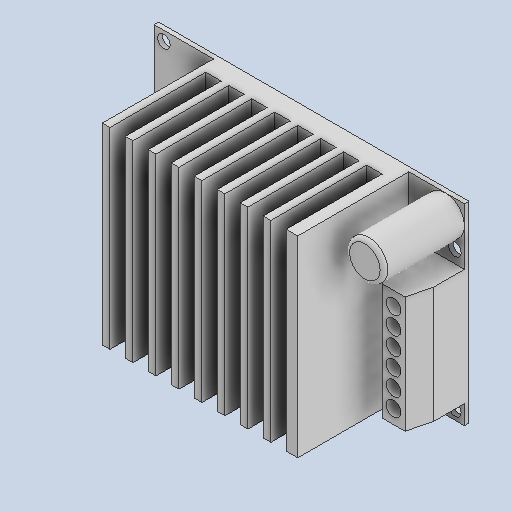
# Autodesk Inventor part: HiLetgoTB6600HG
Saved by Autodesk Inventor 2025.2 (Build 292293000, 293)
## iProperties
Created: 2025-02-08
Part Number: HiLetgoTB6600HG
Material: Generic
Document SubType Name: Modeling
Designer: LattePanda
Density: 1 g/cm^3
Appearance: Default
Author: LattePanda
Autodesk Inventor part; units mm, degrees
ref_plane "YZ Plane" through (0, 0, 0) normal (1, 0, 0) x (0, 1, 0)
ref_plane "XZ Plane" through (0, 0, 0) normal (0, 1, 0) x (-1, 0, 0)
ref_plane "XY Plane" through (0, 0, 0) normal (0, 0, 1) x (1, 0, 0)
sketch "Sketch1" plane through (0, 0, 0) normal (0, 0, 1) x (1, 0, 0)
  line L0 (-40.485, -25.075) -> (40.485, -25.075)
  line L1 (40.485, -25.075) -> (40.485, 25.075)
  line L2 (40.485, 25.075) -> (-40.485, 25.075)
  line L3 (-40.485, 25.075) -> (-40.485, -25.075)
  line L4 (-40.485, -25.075) -> (40.485, 25.075) construction
  line L5 (40.485, -25.075) -> (-40.485, 25.075) construction
  circle A0 centre (-37.975, 22.565) radius 1.65
  line L6 (-39.625, 24.215) -> (-36.325, 24.215) construction
  line L7 (-36.325, 24.215) -> (-36.325, 20.915) construction
  line L8 (-36.325, 20.915) -> (-39.625, 20.915) construction
  line L9 (-39.625, 20.915) -> (-39.625, 24.215) construction
  line L10 (-39.625, 24.215) -> (-36.325, 20.915) construction
  line L11 (-36.325, 24.215) -> (-39.625, 20.915) construction
  line L12 (-40.485, 0) -> (40.485, 0) construction
  line L13 (0, 25.075) -> (0, -25.075) construction
  circle A1 centre (-37.975, -22.565) radius 1.65
  line L14 (0, -25.075) -> (0, 25.075) construction
  circle A2 centre (37.975, 22.565) radius 1.65 construction
  circle A3 centre (37.975, -22.565) radius 1.65
  line L15 (37.975, 25.075) -> (37.975, 13.575) construction
  circle A4 centre (37.975, 13.575) radius 1.65
  point P0 (0, 0)
  dimension "d0" = 80.97
  dimension "d1" = 50.15
  dimension "d2" = 3.3
  dimension "d3" = 0.86
  dimension "d4" = 0.86
  dimension "d10" = 11.5
  constraints: 32 end point, 8 midpoint, 5 centre point, 5 symmetric about line, 4 parallel, 2 horizontal, 2 perpendicular, 2 tangent, 1 coincident, 1 equal radius, 1 point on line, 1 vertical, 3 other
  measures "d0" distance of L1.end L2.end
  measures "d1" distance of L2.end L0.start
  measures "d2" diameter of A0
  measures "d3" distance between parallel lines of L2 L6
  measures "d4" distance between parallel lines of L3 L9
  measures "d10" distance of L15.start L15.end
extrude "Extrusion1" add sketch "Sketch1" along normal blind 1.17
sketch "Sketch2" plane through (0, 0, 1.17) normal (0, 0, 1) x (1, 0, 0)
  line L0 (40.485, -25.075) -> (40.485, 25.075) projected
  line L1 (40.485, -20.075) -> (30.485, -20.075)
  line L2 (30.485, -20.075) -> (30.485, 10.275)
  line L3 (30.485, 10.275) -> (40.485, 10.275)
  line L4 (40.485, 10.275) -> (40.485, -20.075)
  line L5 (-40.485, -25.075) -> (40.485, -25.075) projected
  point P0 (0, 0)
  dimension "d7" = 5
  dimension "d8" = 30.35
  dimension "d9" = 10
  constraints: 8 end point, 2 parallel, 1 horizontal, 1 perpendicular, 1 point on line
  measures "d7" distance between parallel lines of L5 L1
  measures "d8" distance of L1.end L2.end
  measures "d9" distance between parallel lines of L0 L2
extrude "Extrusion2" add sketch "Sketch2" along normal blind 14
sketch "Sketch3" plane through (0, 0, 1.17) normal (0, 0, 1) x (1, 0, 0)
  line L0 (40.485, 10.275) -> (40.485, 25.075) construction
  line L1 (40.485, 25.075) -> (-40.485, 25.075) construction
  circle A0 centre (35.485, 20.075) radius 5
  point P0 (0, 0)
  dimension "d13" = 10
  constraints: 2 tangent, 1 centre point
  measures "d13" diameter of A0
extrude "Extrusion3" add sketch "Sketch3" along normal blind 21
fillet "Fillet1" radius 1 1 edges at (30.485, 20.075, 22.17)
sketch "Sketch4" plane through (30.485, -20.075, 1.17) normal (0, -1, 0) x (1, 0, 0)
  line L0 (0, 14) -> (10, 14) construction
  line L1 (0, 0) -> (0, 14) projected
  line L2 (10, 0) -> (10, 14) projected
  line L3 (10, 14) -> (0, 14) projected
  line L4 (2.5, 14) -> (8.5, 14)
  line L5 (10, 8) -> (8.5, 14)
  line L6 (2.5, 14) -> (0, 8)
  line L7 (10, 8) -> (0, 8) construction
  point P0 (-30.485, -1.17)
  dimension "d17" = 6
  dimension "d18" = 6
  dimension "d19" = 1.5
  constraints: 8 end point, 4 point on line, 1 horizontal
  measures "d17" distance between parallel lines of L7 L0
  measures "d18" distance of L4.end L4.start
  measures "d19" distance of L0.end L4.end
extrude "Extrusion4" cut sketch "Sketch4" against normal up to surface (30.35 mm away)
sketch "Sketch5" plane through (0, 0, 15.17) normal (0, 0, 1) x (1, 0, 0)
  line L0 (38.985, 10.275) -> (32.985, 10.275) construction
  line L1 (35.985, 10.275) -> (35.985, -20.075) construction
  line L2 (32.985, -20.075) -> (38.985, -20.075) construction
  line L3 (35.985, -20.075) -> (35.985, 10.275) construction
  circle A0 centre (35.985, 6.6536) radius 1.925
  circle A1 centre (35.985, 2.0321) radius 1.925
  circle A2 centre (35.985, -2.5893) radius 1.925
  circle A3 centre (35.985, -7.2107) radius 1.925
  circle A4 centre (35.985, -11.8321) radius 1.925
  circle A5 centre (35.985, -16.4536) radius 1.925
  point P0 (0, 0)
  dimension "d22" = 3.85
  dimension "d23" = 4.6214
  dimension "d24" = 4.6214
  dimension "d25" = 4.6214
  dimension "d26" = 4.6214
  dimension "d27" = 4.6214
  dimension "d28" = 3.6214
  dimension "d29" = 3.6214
  constraints: 6 centre point, 6 point on line, 5 equal radius, 4 end point, 2 midpoint, 1 collinear
  measures "d22" diameter of A0
  measures "d23" distance of A1.centre A0.centre
  measures "d24" distance of A2.centre A1.centre
  measures "d25" distance of A3.centre A2.centre
  measures "d26" distance of A4.centre A3.centre
  measures "d27" distance of A4.centre A5.centre
  measures "d28" distance from line of A0.centre L0
  measures "d29" distance from line of L2 A5.centre
extrude "Extrusion5" cut sketch "Sketch5" against normal blind 3.85
sketch "Sketch6" plane through (0, 0, 1.17) normal (0, 0, 1) x (1, 0, 0)
  line L0 (-25.015, 25.075) -> (25.985, 25.075)
  line L1 (25.985, 25.075) -> (25.985, -25.075)
  line L2 (25.985, -25.075) -> (-25.015, -25.075)
  line L3 (-25.015, -25.075) -> (-25.015, 25.075)
  line L4 (40.485, -25.075) -> (40.485, -20.075) projected
  line L5 (35.485, 25.075) -> (-40.485, 25.075) projected
  line L6 (-40.485, -25.075) -> (40.485, -25.075) projected
  point P0 (0, 0)
  dimension "d32" = 14.5
  dimension "d33" = 51
  constraints: 8 end point, 2 collinear, 2 parallel, 1 horizontal, 1 perpendicular
  measures "d32" distance between parallel lines of L4 L1
  measures "d33" distance between parallel lines of L1 L3
extrude "Extrusion6" add sketch "Sketch6" along normal blind 29
sketch "Sketch7" plane through (0, 0, 30.17) normal (0, 0, 1) x (1, 0, 0)
  line L0 (25.985, 25.075) -> (-25.015, 25.075) projected
  line L1 (-25.015, -25.075) -> (25.985, -25.075) projected
  line L2 (22.985, 25.075) -> (18.985, 25.075)
  line L3 (18.985, 25.075) -> (18.985, -25.075)
  line L4 (18.985, -25.075) -> (22.985, -25.075)
  line L5 (22.985, -25.075) -> (22.985, 25.075)
  line L6 (25.985, -25.075) -> (25.985, 25.075) projected
  line L7 (16.985, 25.075) -> (16.985, -25.075)
  line L8 (12.985, 25.075) -> (12.985, -25.075)
  line L9 (10.985, 25.075) -> (10.985, -25.075)
  line L10 (6.985, 25.075) -> (6.985, -25.075)
  line L11 (4.985, 25.075) -> (4.985, -25.075)
  line L12 (0.985, 25.075) -> (0.985, -25.075)
  line L13 (-1.015, 25.075) -> (-1.015, -25.075)
  line L14 (-5.015, 25.075) -> (-5.015, -25.075)
  line L15 (-7.015, 25.075) -> (-7.015, -25.075)
  line L16 (-11.015, 25.075) -> (-11.015, -25.075)
  line L17 (-13.015, 25.075) -> (-13.015, -25.075)
  line L18 (-17.015, 25.075) -> (-17.015, -25.075)
  line L19 (-19.015, 25.075) -> (-19.015, -25.075)
  line L20 (-23.015, 25.075) -> (-23.015, -25.075)
  point P0 (0, 0)
  dimension "d36" = 3
  dimension "d37" = 4
  dimension "d38" = 2
  dimension "d39" = 4
  dimension "d40" = 2
  dimension "d41" = 4
  dimension "d42" = 2
  dimension "d43" = 4
  dimension "d44" = 2
  dimension "d45" = 4
  dimension "d46" = 2
  dimension "d47" = 4
  dimension "d48" = 2
  dimension "d49" = 4
  dimension "d50" = 2
  dimension "d51" = 4
  constraints: 36 end point, 12 vertical, 4 parallel, 1 horizontal, 1 perpendicular, 32 other
  measures "d36" distance between parallel lines of L6 L5
  measures "d37" distance between parallel lines of L5 L3
  measures "d38" distance between parallel lines of L3 L7
  measures "d39" distance between parallel lines of L7 L8
  measures "d40" distance between parallel lines of L8 L9
  measures "d41" distance between parallel lines of L10 L9
  measures "d42" distance between parallel lines of L11 L10
  measures "d43" distance between parallel lines of L12 L11
  measures "d44" distance between parallel lines of L13 L12
  measures "d45" distance between parallel lines of L14 L13
  measures "d46" distance between parallel lines of L15 L14
  measures "d47" distance between parallel lines of L16 L15
  measures "d48" distance between parallel lines of L17 L16
  measures "d49" distance between parallel lines of L18 L17
  measures "d50" distance between parallel lines of L19 L18
  measures "d51" distance between parallel lines of L20 L19
extrude "Extrusion7" cut sketch "Sketch7" against normal blind 25 contours L5 L1 L3 L0 | L7 L1 L8 L0 | L9 L1 L10 L0 | L11 L1 L12 L0 | L13 L1 L14 L0 | L15 L1 L16 L0 | L17 L1 L18 L0 | L19 L1 L20 L0
sketch "Sketch8" plane through (0, 0, 1.17) normal (0, 0, 1) x (1, 0, 0)
  line L0 (32.985, -20.075) -> (38.985, -20.075) projected
  line L1 (30.485, -20.075) -> (-40.485, -20.075) construction
  line L2 (-40.485, 25.075) -> (-40.485, -25.075) projected
  line L3 (-40.485, -20.075) -> (-30.485, -20.075)
  line L4 (-30.485, -20.075) -> (-30.485, -0.075)
  line L5 (-30.485, -0.075) -> (-40.485, -0.075)
  line L6 (-40.485, -0.075) -> (-40.485, -20.075)
  line L7 (40.485, 10.275) -> (40.485, -20.075) projected
  line L8 (30.485, -20.075) -> (30.485, 10.275) projected
  point P0 (0, 0)
  point P1 (-30.485, -10.075)
  dimension "d54" = 20
  dimension "d55" = 10
  dimension "d56" = 10
  constraints: 10 end point, 2 horizontal, 2 parallel, 1 midpoint, 1 perpendicular, 1 point on line
  measures "d54" distance of L3.end L4.end
  measures "d55" distance between parallel lines of L7 L8
  measures "d56" distance from line of point (-30.485, -10.075) L2
extrude "Extrusion8" add sketch "Sketch8" along normal up to surface (14 mm away)
sketch "Sketch10" plane through (-40.485, -20.075, 1.17) normal (0, -1, 0) x (1, 0, 0)
  line L0 (10, 14) -> (0, 14) projected
  line L1 (2.6888, 14) -> (7.5, 14)
  line L2 (10, 0) -> (10, 14) projected
  line L3 (10, 8) -> (7.5, 14)
  line L4 (0, 0) -> (0, 14) projected
  line L5 (1.5, 14) -> (0, 8)
  line L6 (73.47, 14) -> (79.47, 14) projected
  line L7 (80.97, 8) -> (79.47, 14) projected
  line L8 (73.47, 14) -> (70.97, 8) projected
  point P0 (40.485, -1.17)
  point P1 (76.47, 14)
  dimension "d59" = 1.5
  dimension "d60" = 1.5
  dimension "d61" = 2.5
  dimension "d62" = 2.5
  dimension "d63" = 6
  dimension "d64" = 6
  dimension "d65" = 6
  constraints: 6 end point, 5 point on line, 1 midpoint
  measures "d59" horizontal distance of L7.start L6.end
  measures "d60" distance of L0.end L5.start
  measures "d61" horizontal distance of L8.end L6.start
  measures "d62" distance from line of L2 L1.end
  measures "d63" vertical distance of L7.start point (76.47, 14)
  measures "d64" vertical distance of L3.start L1.end
  measures "d65" vertical distance of L5.start L5.end
extrude "Extrusion9" cut sketch "Sketch10" against normal up to surface (20 mm away)
sketch "Sketch11" plane through (-38.985, -0.075, 15.17) normal (0, 0, 1) x (1, 0, 0)
  line L0 (0, 0) -> (6, 0) construction
  line L1 (6, -20) -> (0, -20) construction
  line L2 (3, 0) -> (3, -20) construction
  circle A0 centre (3, -3) radius 1.925
  circle A1 centre (3, -7.6667) radius 1.925
  circle A2 centre (3, -12.3333) radius 1.925
  circle A3 centre (3, -17) radius 1.925
  circle A4 centre (74.97, 6.7286) radius 1.925 projected
  point P0 (38.985, 0.075)
  dimension "d68" = 3
  dimension "d69" = 3
  dimension "d70" = 4.6667
  dimension "d71" = 4.6667
  dimension "d73" = 4.6667
  constraints: 4 centre point, 4 equal radius, 4 point on line, 2 end point, 2 midpoint
  measures "d68" distance from line of L0 A0.centre
  measures "d69" distance from line of L1 A3.centre
  measures "d70" distance of A1.centre A0.centre
  measures "d71" distance of A2.centre A1.centre
  measures "d73" distance of A3.centre A2.centre
extrude "Extrusion10" cut sketch "Sketch11" against normal blind 10 contours A0 | A1 | A2 | A3
equation "\"d24\" = d23"
equation "\"d25\" = d23"
equation "\"d26\" = d23"
equation "\"d27\" = d23"
equation "\"d30\" = d22"
equation "\"d39\" = d37"
equation "\"d40\" = d38"
equation "\"d41\" = d37"
equation "\"d42\" = d38"
equation "\"d43\" = d37"
equation "\"d44\" = d38"
equation "\"d45\" = d37"
equation "\"d46\" = d38"
equation "\"d47\" = d37"
equation "\"d48\" = d38"
equation "\"d49\" = d37"
equation "\"d50\" = d38"
equation "\"d51\" = d37"
equation "\"d56\" = d55"
equation "\"d60\" = d59"
equation "\"d62\" = d61"
equation "\"d64\" = d63"
equation "\"d65\" = d63"
equation "\"d71\" = d70"
equation "\"d73\" = d70"
body "Solid1"
